Autodesk Inventor part; units mm, degrees
(part 2 of 2)
sketch "Sketch20" plane through (0, -205.7831, -50.0038) normal (0, -1, 0) x (1, 0, 0)
  circle A0 centre (18.288, 75.425) radius 2.032
  line L0 (20.32, 98.425) -> (0, 98.425) projected
  line L1 (20.32, 95.25) -> (20.32, 63.2968) projected
  point P0 (0, 50.0038)
  dimension "d126" = 4.064
  dimension "d127" = 23
  dimension "d128" = 2.032
  constraints: 1 centre point
  measures "d126" diameter of A0
  measures "d127" distance from line of L0 A0.centre
  measures "d128" distance from line of L1 A0.centre
extrude "Extrusion12" cut sketch "Sketch20" against normal blind 13.97
sketch "Sketch21" plane through (6.35, 0, 0) normal (1, 0, 0) x (0, 0, -1)
  circle A0 centre (-38.2612, -35.6031) radius 1.9939 projected
  arc A1 (-36.9446, -43.9621) -> (-35.2132, -41.1342) centre (-38.3882, -41.1342) ccw
  line L0 (-36.9446, -43.9621) -> (-40.0971, -45.5714)
  arc A2 (-40.0971, -45.5714) -> (-41.4581, -46.9108) centre (-38.6535, -48.3993) ccw
  line L1 (-41.0534, -42.2715) -> (-41.1957, -42.6431)
  line L2 (-35.2132, -31.0115) -> (-35.2132, -41.1342)
  line L3 (-41.4581, -46.9108) -> (-42.0712, -48.0662)
  arc A3 (-35.2132, -31.0115) -> (-36.9446, -28.1837) centre (-38.3882, -31.0115) ccw
  line L4 (-36.9446, -28.1837) -> (-40.0971, -26.5743)
  arc A4 (-41.4581, -25.2349) -> (-40.0971, -26.5743) centre (-38.6535, -23.7465) ccw
  line L5 (-41.4581, -25.2349) -> (-42.0712, -24.0796)
  line L6 (-42.0712, -24.0796) -> (-42.0712, -48.0662)
  line L7 (-42.0712, 41.2319) -> (-42.0712, -196.2581) projected
  circle A5 centre (-38.2612, -35.6031) radius 1.9939
  line L8 (46.8288, 41.2319) -> (46.8288, -196.2581) projected
  line L9 (46.8288, -28.4911) -> (46.8288, -42.7151)
  line L10 (39.9708, -40.77) -> (39.9708, -30.4361)
  circle A6 centre (43.0188, -35.6031) radius 1.9939 projected
  circle A7 centre (43.0188, -35.6031) radius 1.9939
  line L11 (41.7036, -27.6076) -> (44.8532, -26.0017)
  line L12 (46.2148, -24.6629) -> (46.8288, -23.5074)
  line L13 (41.7036, -43.5986) -> (44.8532, -45.2045)
  line L14 (46.2148, -46.5432) -> (46.8288, -47.6988)
  arc A8 (41.7036, -27.6076) -> (39.9708, -30.4361) centre (43.1458, -30.4361) ccw
  arc A9 (44.8532, -26.0017) -> (46.2148, -24.6629) centre (43.411, -23.1731) ccw
  arc A10 (39.9708, -40.77) -> (41.7036, -43.5986) centre (43.1458, -40.77) ccw
  arc A11 (46.2148, -46.5432) -> (44.8532, -45.2045) centre (43.411, -48.033) ccw
  line L15 (46.8288, -23.5074) -> (46.8288, -47.6988)
  point P0 (0, 0)
  point P1 (-37.8414, -35.6031)
  point P2 (-40.9888, -46.0266)
  point P3 (-37.853, -42.7151)
  point P4 (-37.853, -28.4911)
  point P5 (-40.9888, -26.1192)
  point P6 (-42.0712, -47.4903)
  point P7 (43.3998, -28.4911)
  point P8 (45.745, -25.547)
  point P9 (45.745, -45.6592)
  dimension "d135" = 14.224
  dimension "d136" = 2.0396
  dimension "d137" = 2.0396
  dimension "d138" = 145
  dimension "d139" = 145
  dimension "d140" = 117.044
  dimension "d141" = 117.044
  dimension "d142" = 3.175
  dimension "d143" = 6.858
  dimension "d144" = 7.112
  dimension "d146" = 3.1525
  dimension "d147" = 0
  dimension "d148" = 0
  dimension "d149" = 3.9878
  dimension "d153" = 6.858
  dimension "d154" = 2.0396
  dimension "d155" = 145
  dimension "d156" = 2.0396
  dimension "d157" = 145
  dimension "d158" = 3.175
  dimension "d159" = 3.1496
  dimension "d160" = 3.1496
  constraints: 28 end point, 16 point on circle, 16 tangent, 11 point on line, 10 centre point, 7 equal radius, 2 coincident, 1 collinear, 1 parallel, 1 vertical
  measures "d135" distance of point (-37.853, -42.715) point (-37.853, -28.491)
  measures "d136" vertical distance of point (-40.989, -26.119) L6.start
  measures "d137" vertical distance of point (-40.989, -46.027) L3.end
  measures "d138" angle of L3 L0
  measures "d139" angle of L5 L4
  measures "d140" angle of L2 L4
  measures "d141" angle of L0 L2
  measures "d142" radius of A3
  measures "d143" distance between parallel lines of L6 L2
  measures "d144" distance of point (-37.853, -28.491) point (-37.841, -35.603)
  measures "d146" horizontal distance of L4.start L4.end
  measures "d147" distance between parallel lines of L7 L6
  measures "d148" vertical distance of A0.centre point (-37.841, -35.603)
  measures "d149" diameter of A0
  measures "d153" distance between parallel lines of L10 L9
  measures "d154" vertical distance of point (45.745, -25.547) L12.end
  measures "d155" angle of L11 L12
  measures "d156" vertical distance of point (45.745, -45.659) L14.end
  measures "d157" angle of L14 L13
  measures "d158" radius of A8
  measures "d159" horizontal distance of L11.start L11.end
  measures "d160" horizontal distance of L13.start L13.end
extrude "Extrusion13" add sketch "Sketch21" along normal blind 8.89
fillet "Fillet6" radius 0.508 11 edges at (16.002, 50.7569, -20.9208) (11.684, 50.7569, -3.1357) (16.002, 50.7569, 14.6493) (18.161, -47.4903, 48.4212) (16.002, -51.4908, 48.4212) (18.161, -55.4913, 48.4212) (19.7104, -205.7831, 13.293) (18.2245, -205.7831, 12.293) (17.3482, -205.7831, 8.2892) (18.2245, -205.7831, 4.2854) (19.7104, -205.7831, 3.2854)
body "Solid1"
